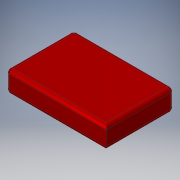
# Autodesk Inventor part: LiPo_Akku
Saved by Autodesk Inventor 2017.3 (Build 213257000, 257)
## iProperties
Part Number: LiPo_Akku
Material: Generisch
Document SubType Name: Modeling
Designer: Enno
Density: 1 g/cm^3
Appearance: Vorgabe
Author: Enno
Autodesk Inventor part; units mm, degrees
ref_plane "YZ Plane" through (0, 0, 0) normal (1, 0, 0) x (0, 1, 0)
ref_plane "XZ Plane" through (0, 0, 0) normal (0, 1, 0) x (-1, 0, 0)
ref_plane "XY Plane" through (0, 0, 0) normal (0, 0, 1) x (1, 0, 0)
sketch "Skizze1" plane through (0, 0, 0) normal (0, 0, 1) x (1, 0, 0)
  line L0 (0, 0) -> (28, 0)
  line L1 (28, 0) -> (28, 19)
  line L2 (28, 19) -> (0, 19)
  line L3 (0, 19) -> (0, 0)
  dimension "d0" = 28
  dimension "d1" = 19
  constraints: 8 end point, 2 parallel, 1 horizontal, 1 perpendicular
  measures "d0" distance of L2.end L1.end
  measures "d1" distance between parallel lines of L0 L2
extrude "Extrusion1" add sketch "Skizze1" along normal blind 6
fillet "Rundung1" radius 1 1 edges at (14, 19, 6)
fillet "Rundung2" radius 1 12 edges at (0, 9, 6) (0, 18.7071, 5.7071) (0, 19, 2.5) (14, 0, 6) (28, 18.7071, 5.7071) (28, 19, 2.5) (28, 9, 6) (0, 9.5, 0) (0, 0, 3) (14, 0, 0) (28, 9.5, 0) (14, 19, 0)
